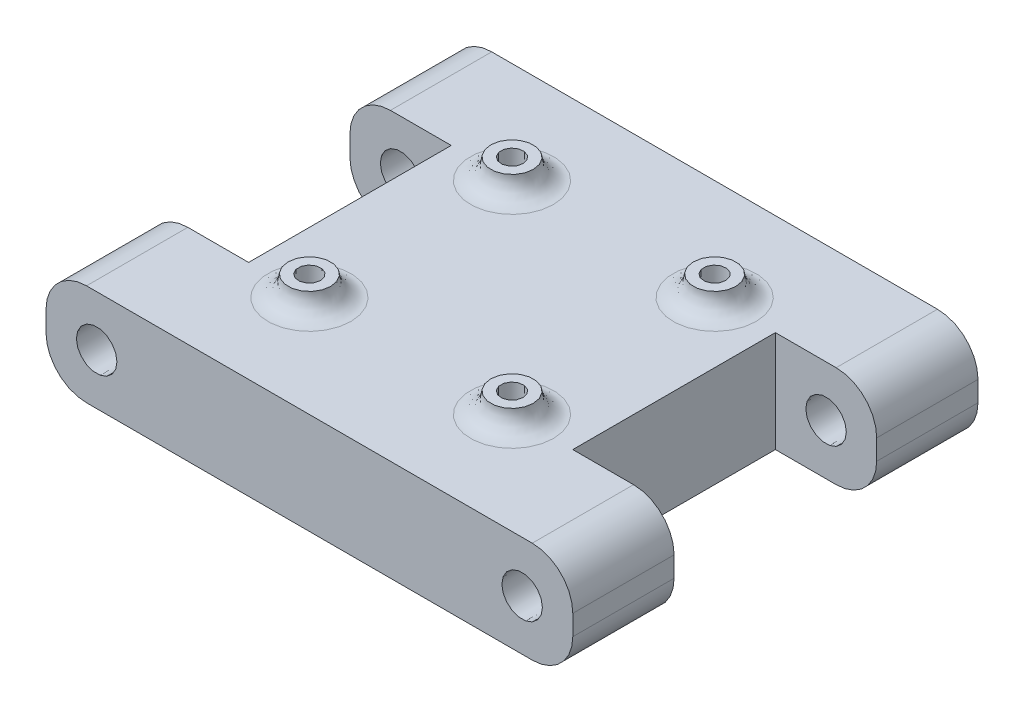
# Autodesk Inventor part: arm
Saved by Autodesk Inventor 2021 (Build 250183000, 183)
## iProperties
Created: 2020-12-29
Part Number: arm
Material: Generic
Document SubType Name: Modeling
Designer: Tomasz
Density: 1 g/cm^3
Appearance: Default
Author: Tomasz
Autodesk Inventor part; units mm, degrees
ref_plane "YZ Plane" through (0, 0, 0) normal (1, 0, 0) x (0, 1, 0)
ref_plane "XZ Plane" through (0, 0, 0) normal (0, 1, 0) x (-1, 0, 0)
ref_plane "XY Plane" through (0, 0, 0) normal (0, 0, 1) x (1, 0, 0)
sketch "arm_sketch" plane through (0, 0, 0) normal (0, 1, 0) x (-1, 0, 0)
  line L0 (0, -40) -> (-32, -40)
  line L1 (-32, -40) -> (-32, 0) construction
  line L2 (-32, 0) -> (0, 0)
  line L3 (0, 0) -> (0, -40) construction
  line L4 (0, -30) -> (-32, -30) construction
  line L5 (-32, -30) -> (-32, -10)
  line L6 (-32, -10) -> (0, -10) construction
  line L7 (0, -10) -> (0, -30)
  line L8 (-32, -40) -> (-42, -40)
  line L9 (-42, -40) -> (-42, -30)
  line L10 (-42, -30) -> (-32, -30)
  line L11 (-32, -30) -> (-32, -40) construction
  line L12 (0, -20) -> (-32, -20) construction
  line L13 (-16, -40) -> (-16, 0) construction
  line L14 (-32, 0) -> (-42, 0)
  line L15 (-42, 0) -> (-42, -10)
  line L16 (-42, -10) -> (-32, -10)
  line L17 (-32, -10) -> (-32, 0) construction
  line L18 (0, -40) -> (10, -40)
  line L19 (10, -40) -> (10, -30)
  line L20 (10, -30) -> (0, -30)
  line L21 (0, -30) -> (0, -40) construction
  line L22 (0, -10) -> (0, 0) construction
  line L23 (0, 0) -> (10, 0)
  line L24 (10, 0) -> (10, -10)
  line L25 (10, -10) -> (0, -10)
  circle A0 centre (-6, -30) radius 1.1
  circle A1 centre (-6, -10) radius 1.1
  circle A2 centre (-26, -30) radius 1.1
  circle A3 centre (-26, -10) radius 1.1
  point P0 (0, -10)
  point P1 (0, -30)
  point P2 (0, -10)
  dimension "d0" = 32
  dimension "d1" = 40
  dimension "d2" = 20
  dimension "d3" = 10
  dimension "d4" = 10
  dimension "d79" = 2.2
  dimension "d82" = 20
  dimension "d85" = 20
  dimension "d88" = 20
  dimension "d89" = 20
  constraints: 52 end point, 13 symmetric about line, 6 parallel, 4 centre point, 4 horizontal, 4 midpoint, 3 perpendicular, 2 coincident, 2 point on line, 1 vertical, 6 other
  measures "d0" distance of L1.end L2.end
  measures "d1" distance of L0.end L1.end
  measures "d2" distance between parallel lines of L6 L4
  measures "d3" distance between parallel lines of L6 L2
  measures "d4" distance of L9.end L10.end
  measures "d79" diameter of A0
  measures "d82" distance of A0.centre A1.centre
  measures "d85" distance of A0.centre A2.centre
  measures "d88" diameter of A0.centre L12
  measures "d89" diameter of A0.centre L13
extrude "arm" add sketch "arm_sketch" along normal blind 10
sketch "arm_holes_sketch" plane through (-10, 0, 0) normal (0, 0, 1) x (1, 0, 0)
  line L0 (10, 0) -> (10, 10) construction
  line L1 (42, 0) -> (42, 10) construction
  line L2 (52, 0) -> (52, 10) construction
  line L3 (0, 0) -> (0, 10) construction
  circle A0 centre (5, 5) radius 2
  circle A1 centre (47, 5) radius 2
  dimension "d42" = 4
  dimension "d43" = 4
  dimension "d44" = 10
  dimension "d45" = 10
  dimension "d46" = 10
  dimension "d47" = 10
  dimension "d48" = 5
  dimension "d49" = 5
  dimension "d50" = 5
  dimension "d51" = 5
  constraints: 2 centre point
  measures "d42" diameter of A0
  measures "d43" diameter of A1
  measures "d44" distance of L0.start L0.end
  measures "d45" distance between parallel lines of L0 L3
  measures "d46" distance of L1.start L1.end
  measures "d47" distance between parallel lines of L2 L1
  measures "d48" distance from line of L1 A1.centre
  measures "d49" horizontal distance of L1.start A1.centre
  measures "d50" distance from line of L0 A0.centre
  measures "d51" horizontal distance of L0.start A0.centre
extrude "arm_holes" cut sketch "arm_holes_sketch" against normal through all
fillet "round_rot_edge" radius 4 8 edges at (42, 10, -5) (42, 0, -5) (42, 0, -35) (42, 10, -35) (-10, 10, -5) (-10, 10, -35) (-10, 0, -5) (-10, 0, -35)
sketch "Sketch6" plane through (0, 10, 0) normal (0, 1, 0) x (1, 0, 0)
  circle A0 centre (6, 30) radius 1.1 projected
  circle A1 centre (26, 30) radius 1.1 projected
  circle A2 centre (26, 10) radius 1.1 projected
  circle A3 centre (6, 10) radius 1.1 projected
  circle A4 centre (6, 30) radius 2.1
  line L0 (6, 30) -> (26, 30) construction
  line L1 (6, 30) -> (6, 10) construction
  circle A5 centre (26, 30) radius 2.1
  circle A6 centre (6, 10) radius 2.1
  circle A7 centre (26, 10) radius 2.1
  point P0 (0, 0)
  dimension "d90" = 20
  dimension "d91" = 20
  dimension "d92" = 4.2
  dimension "d95" = 20
  dimension "d98" = 20
  constraints: 4 centre point, 4 end point, 2 horizontal, 2 vertical, 1 coincident, 6 other
  measures "d90" distance of L0.end A0.centre
  measures "d91" distance of L1.end A0.centre
  measures "d92" diameter of A4
  measures "d95" distance of L0.start A5.centre
  measures "d98" distance of L0.start A6.centre
extrude "Extrusion6" add sketch "Sketch6" along normal blind 2
fillet "Fillet4" radius 2 4 edges at (3.9, 10, -30) (23.9, 10, -30) (3.9, 10, -10) (23.9, 10, -10)
equation "\"d3\" = 0.5 * d1 - 0.5 * d2"
equation "\"d79\" = hole"
equation "\"d88\" = d82"
equation "\"d89\" = d85"
equation "\"d42\" = arm_rod_diam"
equation "\"d43\" = arm_rod_diam"
equation "\"d48\" = 0.5 * d47"
equation "\"d49\" = 0.5 * d46"
equation "\"d50\" = 0.5 * d45"
equation "\"d51\" = 0.5 * d44"
equation "\"d37\" = arm_rod_diam"
equation "\"d95\" = d90"
equation "\"d98\" = d91"
equation "\"arm_rod_diam\" = 4"
equation "\"hole\" = 2.2"
body "Solid1"
